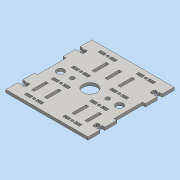
# Autodesk Inventor part: Y-Anchor_Front
Saved by Autodesk Inventor 2016 SP1 (Build 200210100, 210)
## iProperties
Created: 2015-12-01
Part Number: Y-Anchor_Front
Material: Generic
Document SubType Name: Modeling
Designer: Mohamed A.
Density: 1 g/cm^3
Appearance: Default
Author: Mohamed A.
Autodesk Inventor part; units mm, degrees
ref_plane "YZ Plane" through (0, 0, 0) normal (1, 0, 0) x (0, 1, 0)
ref_plane "XZ Plane" through (0, 0, 0) normal (0, 1, 0) x (-1, 0, 0)
ref_plane "XY Plane" through (0, 0, 0) normal (0, 0, 1) x (1, 0, 0)
sketch "Sketch1" plane through (0, 0, 0) normal (0, 0, 1) x (1, 0, 0)
  circle A0 centre (0, 0) radius 7.5
  circle A1 centre (18.5, 0) radius 2.25
  circle A2 centre (-18.5, 0) radius 2.25
  circle A3 centre (30.8333, 0) radius 3.9
  circle A4 centre (-30.8333, 0) radius 3.9
  line L0 (-51.1513, 0) -> (71.4472, 0) construction
  line L1 (15.8333, -16.9294) -> (39.8333, -16.9294) construction
  line L2 (39.8333, -16.9294) -> (39.8333, -31.9294) construction
  line L3 (39.8333, -31.9294) -> (15.8333, -31.9294) construction
  line L4 (15.8333, -31.9294) -> (15.8333, -16.9294) construction
  arc A5 (-21.25, 4.9867) -> (-24, 2.1319) centre (-18.93, 0) ccw construction
  line L5 (-24, -2.1319) -> (-24, 2.1319) construction
  arc A6 (-24, -2.1319) -> (-21.25, -4.9867) centre (-18.93, 0) ccw construction
  line L6 (-10.125, -8.9294) -> (-21.25, -4.9867) construction
  arc A7 (-10.125, -8.9294) -> (10.125, -8.9294) centre (0, 0) ccw construction
  line L7 (21.25, -4.9867) -> (10.125, -8.9294) construction
  arc A8 (21.25, -4.9867) -> (24, -2.1319) centre (18.93, 0) ccw construction
  line L8 (24, 2.1319) -> (24, -2.1319) construction
  arc A9 (24, 2.1319) -> (21.25, 4.9867) centre (18.93, 0) ccw construction
  line L9 (10.125, 8.9294) -> (21.25, 4.9867) construction
  arc A10 (10.125, 8.9294) -> (-10.125, 8.9294) centre (0, 0) ccw construction
  line L10 (-21.25, 4.9867) -> (-10.125, 8.9294) construction
  line L11 (0, 50.1847) -> (0, -53.8877) construction
  line L12 (11.0648, -8.9294) -> (17.2667, -8.9294)
  line L13 (28.7685, -8.9294) -> (28.7685, -11.9294)
  line L14 (28.7685, -11.9294) -> (22.5667, -11.9294)
  line L15 (11.0648, -11.9294) -> (11.0648, -8.9294)
  line L16 (27.8333, -15.5254) -> (27.8333, -35.4643) construction
  line L17 (48.9929, -24.4294) -> (9.7408, -24.4294) construction
  line L18 (19.9167, -5.8226) -> (19.9167, -14.0511) construction
  line L19 (64.5029, 29.9529) -> (40.2998, 29.9529) construction
  line L20 (34.8333, 31.4529) -> (34.8333, 28.4529)
  line L21 (35.4333, 32.6029) -> (37.8333, 32.6029)
  line L22 (37.8333, 27.3029) -> (35.4333, 27.3029)
  line L23 (39.8333, 32.6029) -> (42.8333, 32.6029)
  line L24 (42.8333, 27.3029) -> (39.8333, 27.3029)
  line L25 (39.8333, 27.3029) -> (39.8333, 28.4529)
  line L26 (42.8333, 14.9765) -> (42.8333, 27.3029)
  line L27 (42.8333, 32.6029) -> (42.8333, 44.9294)
  line L28 (39.8333, 31.4529) -> (37.8333, 31.4529)
  line L29 (35.4333, 31.4529) -> (34.8333, 31.4529)
  line L30 (34.8333, 28.4529) -> (35.4333, 28.4529)
  line L31 (37.8333, 28.4529) -> (39.8333, 28.4529)
  line L32 (37.8333, 32.6029) -> (37.8333, 31.4529)
  line L33 (37.8333, 28.4529) -> (37.8333, 27.3029)
  line L34 (35.4333, 27.3029) -> (35.4333, 28.4529)
  line L35 (35.4333, 31.4529) -> (35.4333, 32.6029)
  line L36 (39.8333, 32.6029) -> (39.8333, 31.4529)
  line L37 (39.8333, 28.4529) -> (39.8333, 27.3029)
  line L38 (39.8333, 31.4529) -> (39.8333, 32.6029)
  line L39 (42.8333, 14.9765) -> (39.8333, 14.9765)
  line L40 (39.8333, 14.9765) -> (39.8333, -14.9765)
  line L41 (39.8333, -14.9765) -> (42.8333, -14.9765)
  line L42 (34.8333, -31.4529) -> (34.8333, -28.4529)
  line L43 (35.4333, -32.6029) -> (37.8333, -32.6029)
  line L44 (37.8333, -27.3029) -> (35.4333, -27.3029)
  line L45 (39.8333, -32.6029) -> (42.8333, -32.6029)
  line L46 (42.8333, -27.3029) -> (39.8333, -27.3029)
  line L47 (39.8333, -27.3029) -> (39.8333, -28.4529)
  line L48 (42.8333, -14.9765) -> (42.8333, -27.3029)
  line L49 (42.8333, -32.6029) -> (42.8333, -44.9294)
  line L50 (39.8333, -31.4529) -> (37.8333, -31.4529)
  line L51 (35.4333, -31.4529) -> (34.8333, -31.4529)
  line L52 (34.8333, -28.4529) -> (35.4333, -28.4529)
  line L53 (37.8333, -28.4529) -> (39.8333, -28.4529)
  line L54 (37.8333, -32.6029) -> (37.8333, -31.4529)
  line L55 (37.8333, -28.4529) -> (37.8333, -27.3029)
  line L56 (35.4333, -27.3029) -> (35.4333, -28.4529)
  line L57 (35.4333, -31.4529) -> (35.4333, -32.6029)
  line L58 (39.8333, -32.6029) -> (39.8333, -31.4529)
  line L59 (-34.8333, 31.4529) -> (-34.8333, 28.4529)
  line L60 (-35.4333, 32.6029) -> (-37.8333, 32.6029)
  line L61 (-37.8333, 27.3029) -> (-35.4333, 27.3029)
  line L62 (-39.8333, 32.6029) -> (-42.8333, 32.6029)
  line L63 (-42.8333, 27.3029) -> (-39.8333, 27.3029)
  line L64 (-39.8333, 27.3029) -> (-39.8333, 28.4529)
  line L65 (-42.8333, 14.9765) -> (-42.8333, 27.3029)
  line L66 (-42.8333, 32.6029) -> (-42.8333, 44.9294)
  line L67 (-39.8333, 31.4529) -> (-37.8333, 31.4529)
  line L68 (-35.4333, 31.4529) -> (-34.8333, 31.4529)
  line L69 (-34.8333, 28.4529) -> (-35.4333, 28.4529)
  line L70 (-37.8333, 28.4529) -> (-39.8333, 28.4529)
  line L71 (-37.8333, 32.6029) -> (-37.8333, 31.4529)
  line L72 (-37.8333, 28.4529) -> (-37.8333, 27.3029)
  line L73 (-35.4333, 27.3029) -> (-35.4333, 28.4529)
  line L74 (-35.4333, 31.4529) -> (-35.4333, 32.6029)
  line L75 (-39.8333, 32.6029) -> (-39.8333, 31.4529)
  line L76 (-42.8333, 14.9765) -> (-39.8333, 14.9765)
  line L77 (-39.8333, 14.9765) -> (-39.8333, -14.9765)
  line L78 (-39.8333, -14.9765) -> (-42.8333, -14.9765)
  line L79 (-42.8333, -32.6029) -> (-42.8333, -44.9294)
  line L80 (-39.8333, -32.6029) -> (-42.8333, -32.6029)
  line L81 (-39.8333, -32.6029) -> (-39.8333, -31.4529)
  line L82 (-39.8333, -31.4529) -> (-37.8333, -31.4529)
  line L83 (-37.8333, -32.6029) -> (-37.8333, -31.4529)
  line L84 (-35.4333, -32.6029) -> (-37.8333, -32.6029)
  line L85 (-35.4333, -31.4529) -> (-35.4333, -32.6029)
  line L86 (-35.4333, -31.4529) -> (-34.8333, -31.4529)
  line L87 (-34.8333, -31.4529) -> (-34.8333, -28.4529)
  line L88 (-34.8333, -28.4529) -> (-35.4333, -28.4529)
  line L89 (-35.4333, -27.3029) -> (-35.4333, -28.4529)
  line L90 (-37.8333, -27.3029) -> (-35.4333, -27.3029)
  line L91 (-37.8333, -28.4529) -> (-37.8333, -27.3029)
  line L92 (-37.8333, -28.4529) -> (-39.8333, -28.4529)
  line L93 (-39.8333, -27.3029) -> (-39.8333, -28.4529)
  line L94 (-42.8333, -27.3029) -> (-39.8333, -27.3029)
  line L95 (-42.8333, -14.9765) -> (-42.8333, -27.3029)
  line L96 (-42.8333, 44.9294) -> (42.8333, 44.9294)
  line L97 (42.8333, -44.9294) -> (-42.8333, -44.9294)
  line L98 (10.125, -8.9294) -> (-10.125, -8.9294) construction
  line L99 (22.5667, -8.9294) -> (22.5667, -11.9294)
  line L100 (17.2667, -8.9294) -> (17.2667, -11.9294)
  line L101 (22.5667, -8.9294) -> (28.7685, -8.9294)
  line L102 (17.2667, -11.9294) -> (11.0648, -11.9294)
  circle A11 centre (19.9167, -10.4294) radius 1.4
  line L103 (11.0648, -39.9294) -> (17.2667, -39.9294)
  line L104 (28.7685, -39.9294) -> (28.7685, -36.9294)
  line L105 (28.7685, -36.9294) -> (22.5667, -36.9294)
  line L106 (11.0648, -36.9294) -> (11.0648, -39.9294)
  line L107 (22.5667, -39.9294) -> (22.5667, -36.9294)
  line L108 (17.2667, -39.9294) -> (17.2667, -36.9294)
  line L109 (22.5667, -39.9294) -> (28.7685, -39.9294)
  line L110 (17.2667, -36.9294) -> (11.0648, -36.9294)
  circle A12 centre (19.9167, -38.4294) radius 1.4
  line L111 (26.3333, -16.9294) -> (29.3333, -16.9294)
  line L112 (29.3333, -16.9294) -> (29.3333, -31.9294)
  line L113 (29.3333, -31.9294) -> (26.3333, -31.9294)
  line L114 (26.3333, -31.9294) -> (26.3333, -16.9294)
  line L115 (15.8333, -16.9294) -> (12.8333, -16.9294)
  line L116 (12.8333, -16.9294) -> (12.8333, -31.9294)
  line L117 (12.8333, -31.9294) -> (15.8333, -31.9294)
  line L118 (15.8333, -31.9294) -> (15.8333, -16.9294)
  line L119 (-11.0648, -8.9294) -> (-17.2667, -8.9294)
  line L120 (-28.7685, -8.9294) -> (-28.7685, -11.9294)
  line L121 (-28.7685, -11.9294) -> (-22.5667, -11.9294)
  line L122 (-11.0648, -11.9294) -> (-11.0648, -8.9294)
  line L123 (-22.5667, -8.9294) -> (-22.5667, -11.9294)
  line L124 (-17.2667, -8.9294) -> (-17.2667, -11.9294)
  line L125 (-22.5667, -8.9294) -> (-28.7685, -8.9294)
  line L126 (-17.2667, -11.9294) -> (-11.0648, -11.9294)
  circle A13 centre (-19.9167, -10.4294) radius 1.4
  circle A14 centre (-19.9167, -38.4294) radius 1.4
  line L127 (-22.5667, -39.9294) -> (-28.7685, -39.9294)
  line L128 (-22.5667, -39.9294) -> (-22.5667, -36.9294)
  line L129 (-28.7685, -36.9294) -> (-22.5667, -36.9294)
  line L130 (-28.7685, -39.9294) -> (-28.7685, -36.9294)
  line L131 (-11.0648, -39.9294) -> (-17.2667, -39.9294)
  line L132 (-17.2667, -39.9294) -> (-17.2667, -36.9294)
  line L133 (-17.2667, -36.9294) -> (-11.0648, -36.9294)
  line L134 (-11.0648, -36.9294) -> (-11.0648, -39.9294)
  line L135 (-26.3333, -16.9294) -> (-29.3333, -16.9294)
  line L136 (-29.3333, -16.9294) -> (-29.3333, -31.9294)
  line L137 (-29.3333, -31.9294) -> (-26.3333, -31.9294)
  line L138 (-26.3333, -31.9294) -> (-26.3333, -16.9294)
  line L139 (-15.8333, -16.9294) -> (-12.8333, -16.9294)
  line L140 (-12.8333, -16.9294) -> (-12.8333, -31.9294)
  line L141 (-12.8333, -31.9294) -> (-15.8333, -31.9294)
  line L142 (-15.8333, -31.9294) -> (-15.8333, -16.9294)
  line L143 (11.0648, 8.9294) -> (17.2667, 8.9294)
  line L144 (28.7685, 8.9294) -> (28.7685, 11.9294)
  line L145 (28.7685, 11.9294) -> (22.5667, 11.9294)
  line L146 (11.0648, 11.9294) -> (11.0648, 8.9294)
  line L147 (22.5667, 8.9294) -> (22.5667, 11.9294)
  line L148 (17.2667, 8.9294) -> (17.2667, 11.9294)
  line L149 (22.5667, 8.9294) -> (28.7685, 8.9294)
  line L150 (17.2667, 11.9294) -> (11.0648, 11.9294)
  circle A15 centre (19.9167, 10.4294) radius 1.4
  circle A16 centre (19.9167, 38.4294) radius 1.4
  line L151 (22.5667, 39.9294) -> (28.7685, 39.9294)
  line L152 (22.5667, 39.9294) -> (22.5667, 36.9294)
  line L153 (28.7685, 36.9294) -> (22.5667, 36.9294)
  line L154 (28.7685, 39.9294) -> (28.7685, 36.9294)
  line L155 (11.0648, 39.9294) -> (17.2667, 39.9294)
  line L156 (17.2667, 39.9294) -> (17.2667, 36.9294)
  line L157 (17.2667, 36.9294) -> (11.0648, 36.9294)
  line L158 (11.0648, 36.9294) -> (11.0648, 39.9294)
  line L159 (-28.7685, 11.9294) -> (-22.5667, 11.9294)
  line L160 (-28.7685, 8.9294) -> (-28.7685, 11.9294)
  line L161 (-22.5667, 8.9294) -> (-28.7685, 8.9294)
  line L162 (-22.5667, 8.9294) -> (-22.5667, 11.9294)
  circle A17 centre (-19.9167, 10.4294) radius 1.4
  line L163 (-17.2667, 8.9294) -> (-17.2667, 11.9294)
  line L164 (-11.0648, 8.9294) -> (-17.2667, 8.9294)
  line L165 (-11.0648, 11.9294) -> (-11.0648, 8.9294)
  line L166 (-17.2667, 11.9294) -> (-11.0648, 11.9294)
  line L167 (-17.2667, 36.9294) -> (-11.0648, 36.9294)
  line L168 (-11.0648, 36.9294) -> (-11.0648, 39.9294)
  line L169 (-11.0648, 39.9294) -> (-17.2667, 39.9294)
  line L170 (-17.2667, 39.9294) -> (-17.2667, 36.9294)
  circle A18 centre (-19.9167, 38.4294) radius 1.4
  line L171 (-22.5667, 39.9294) -> (-22.5667, 36.9294)
  line L172 (-22.5667, 39.9294) -> (-28.7685, 39.9294)
  line L173 (-28.7685, 39.9294) -> (-28.7685, 36.9294)
  line L174 (-28.7685, 36.9294) -> (-22.5667, 36.9294)
  line L175 (12, 31.9294) -> (-12, 31.9294) construction
  line L176 (-12, 31.9294) -> (-12, 16.9294) construction
  line L177 (-12, 16.9294) -> (12, 16.9294) construction
  line L178 (12, 16.9294) -> (12, 31.9294) construction
  line L179 (-17.778, 24.4294) -> (21.8712, 24.4294) construction
  line L180 (12, 31.9294) -> (15, 31.9294)
  line L181 (15, 31.9294) -> (15, 16.9294)
  line L182 (15, 16.9294) -> (12, 16.9294)
  line L183 (12, 16.9294) -> (12, 31.9294)
  line L184 (-12, 31.9294) -> (-15, 31.9294)
  line L185 (-15, 31.9294) -> (-15, 16.9294)
  line L186 (-15, 16.9294) -> (-12, 16.9294)
  line L187 (-12, 16.9294) -> (-12, 31.9294)
  line L188 (-1.5, 16.9294) -> (1.5, 16.9294)
  line L189 (1.5, 16.9294) -> (1.5, 31.9294)
  line L190 (1.5, 31.9294) -> (-1.5, 31.9294)
  line L191 (-1.5, 31.9294) -> (-1.5, 16.9294)
  point P0 (0, 0)
  point P1 (22.8911, -3.8157)
  dimension "d2" = 4.5
  dimension "d3" = 4.5
  dimension "d4" = 7.8
  dimension "d5" = 7.8
  dimension "d61" = 15
  dimension "d62" = 24
  dimension "d63" = 15
  dimension "d64" = 3
  dimension "d76" = 2.4
  dimension "d79" = 3
  dimension "d81" = 29.9529
  dimension "d82" = 8
  dimension "d83" = 5
  dimension "d84" = 3
  dimension "d85" = 29.9529
  dimension "d87" = 17.7037
  dimension "d88" = 39.8333
  dimension "d89" = 12
  dimension "d90" = 5
  dimension "d92" = 5.3
  dimension "d93" = 2.8
  dimension "d94" = 5
  dimension "d95" = 3
  dimension "d96" = 3
  dimension "d97" = 24
  dimension "d98" = 15
  dimension "d99" = 3
  dimension "d100" = 3
  dimension "d101" = 3
  constraints: 384 end point, 129 symmetric about line, 34 parallel, 20 horizontal, 19 centre point, 19 perpendicular, 15 collinear, 13 point on circle, 10 point on line, 6 vertical, 36 other
  measures "d2" diameter of A1
  measures "d3" diameter of A2
  measures "d4" diameter of A3
  measures "d5" diameter of A4
  measures "d61" diameter of A0
  measures "d62" distance of L2.end L3.end
  measures "d63" distance between parallel lines of L3 L1
  measures "d64" distance of L13.start L13.end
  measures "d76" distance of L22.start L22.end
  measures "d79" distance of L26.start L39.end
  measures "d81" distance of L27.end L26.start
  measures "d82" distance between parallel lines of L26 L20
  measures "d83" distance between parallel lines of L27 L32
  measures "d84" distance between parallel lines of L27 L36
  measures "d85" distance between parallel lines of L41 L39
  measures "d87" distance between parallel lines of L15 L13
  measures "d88" distance between parallel lines of L40 L11
  measures "d89" distance from line of L26 A3.centre
  measures "d90" distance between parallel lines of L1 L14
  measures "d92" distance between parallel lines of L100 L99
  measures "d93" diameter of A11
  measures "d94" distance between parallel lines of L97 L109
  measures "d95" distance of L112.end L113.end
  measures "d96" distance of L117.end L116.end
  measures "d97" distance of L177.end L176.end
  measures "d98" distance of L176.end L175.end
  measures "d99" distance of L181.end L182.end
  measures "d100" distance of L186.end L185.end
  measures "d101" distance of L190.end L189.end
extrude "Extrusion1" add sketch "Sketch1" against normal blind 3
sketch "Sketch4" plane through (0, 0, 0) normal (0, 0, 1) x (1, 0, 0)
  line L0 (40.6667, -26) -> (40.6667, 44.9294)
  line L1 (42.8333, 44.9294) -> (15.7222, 44.9294)
  line L2 (15.7222, 44.9294) -> (15.7222, 41.9294)
  line L3 (15.7222, 41.9294) -> (42.8333, 41.9294)
  line L4 (42.8333, 41.9294) -> (42.8333, 44.9294)
  line L5 (-40.6667, 26) -> (-40.6667, -26)
  line L6 (-40.6667, -26) -> (40.6667, -26)
  line L7 (42.8333, 26) -> (-40.6667, 26) projected
  line L8 (-40.6667, -26) -> (-40.6667, 26)
  line L9 (-40.6667, 26) -> (-13.5556, 26)
  line L10 (-13.5556, 26) -> (-13.5556, 23)
  line L11 (-13.5556, 23) -> (-40.6667, 23)
  line L12 (-40.6667, 23) -> (-40.6667, 26)
  line L13 (40.6667, -26) -> (13.5556, -26)
  line L14 (13.5556, -26) -> (13.5556, -23)
  line L15 (13.5556, -23) -> (40.6667, -23)
  line L16 (40.6667, -23) -> (40.6667, -26)
  line L17 (-40.6667, -26) -> (-13.5556, -26)
  line L18 (-13.5556, -26) -> (-13.5556, -23)
  line L19 (-13.5556, -23) -> (-40.6667, -23)
  line L20 (-40.6667, -23) -> (-40.6667, -26)
  line L21 (42.8333, 44.9294) -> (39.8333, 44.9294)
  line L22 (39.8333, 44.9294) -> (39.8333, 27.5961)
  line L23 (39.8333, 27.5961) -> (42.8333, 27.5961)
  line L24 (42.8333, 27.5961) -> (42.8333, 44.9294)
  line L25 (40.6667, -26) -> (37.6667, -26)
  line L26 (37.6667, -26) -> (37.6667, -8.6667)
  line L27 (37.6667, -8.6667) -> (40.6667, -8.6667)
  line L28 (40.6667, -8.6667) -> (40.6667, -26)
  line L29 (-40.6667, 26) -> (42.8333, 26) projected
  line L30 (-40.6667, 26) -> (-37.6667, 26)
  line L31 (-37.6667, 26) -> (-37.6667, 27.5961)
  line L32 (-37.6667, 27.5961) -> (-40.6667, 27.5961)
  line L33 (-40.6667, 27.5961) -> (-40.6667, 26)
  line L34 (40.6667, -26) -> (-40.6667, -26)
  line L35 (-40.6667, -26) -> (-37.6667, -26)
  line L36 (-37.6667, -26) -> (-37.6667, -8.6667)
  line L37 (-37.6667, -8.6667) -> (-40.6667, -8.6667)
  line L38 (-40.6667, -8.6667) -> (-40.6667, -26)
  line L39 (-40.6667, -26) -> (40.6667, -26) projected
  dimension "d42" = 3
  dimension "d43" = 81.3333
  dimension "d45" = 27.1111
  dimension "d46" = 3
  dimension "d47" = 3
  dimension "d48" = 3
  dimension "d49" = 17.3333
  dimension "d50" = 3
  dimension "d58" = 52
  constraints: 72 end point, 18 parallel, 8 horizontal, 8 perpendicular, 3 collinear, 2 point on line, 3 other
  measures "d42" distance of L2.end L1.end
  measures "d45" distance of L2.end L3.end
  measures "d46" distance of L9.end L10.end
  measures "d47" distance of L13.end L14.end
  measures "d48" distance of L23.end L22.end
  measures "d49" distance between parallel lines of L1 L23
  measures "d50" distance of L31.end L32.end
  measures "d58" distance between parallel lines of L7 L39
extrude "Extrusion2" [suppressed]
sketch "Sketch12" plane through (0, 0, 0) normal (0, 0, 1) x (1, 0, 0)
  circle A0 centre (-30.8333, 0) radius 3.9 projected
  circle A1 centre (30.8333, 0) radius 3.9 projected
  circle A2 centre (-18.5, 0) radius 2.25 projected
  circle A3 centre (18.5, 0) radius 2.25 projected
  line L0 (22.6615, -2.5) -> (25.6615, -2.5)
  line L1 (25.6615, -2.5) -> (25.6615, -17.5)
  line L2 (25.6615, -17.5) -> (22.6615, -17.5)
  line L3 (22.6615, -17.5) -> (22.6615, -2.5)
  line L4 (13.6667, -17.5) -> (10.6667, -17.5)
  line L5 (10.6667, -17.5) -> (10.6667, -2.5)
  line L6 (10.6667, -2.5) -> (13.6667, -2.5)
  line L7 (13.6667, -2.5) -> (13.6667, -17.5)
  line L8 (-13.6667, -2.5) -> (-10.6667, -2.5)
  line L9 (-10.6667, -2.5) -> (-10.6667, -17.5)
  line L10 (-10.6667, -17.5) -> (-13.6667, -17.5)
  line L11 (-13.6667, -17.5) -> (-13.6667, -2.5)
  line L12 (-22.6615, -17.5) -> (-25.6615, -17.5)
  line L13 (-25.6615, -17.5) -> (-25.6615, -2.5)
  line L14 (-25.6615, -2.5) -> (-22.6615, -2.5)
  line L15 (-22.6615, -2.5) -> (-22.6615, -17.5)
  point P0 (0, 0)
  constraints: 32 end point, 8 horizontal, 8 vertical, 16 other
extrude "Extrusion9" [suppressed]
equation "\"d45\" = 0.333333 * d43"
equation "\"d49\" = 0.333333 * d58"
body "Solid1"
